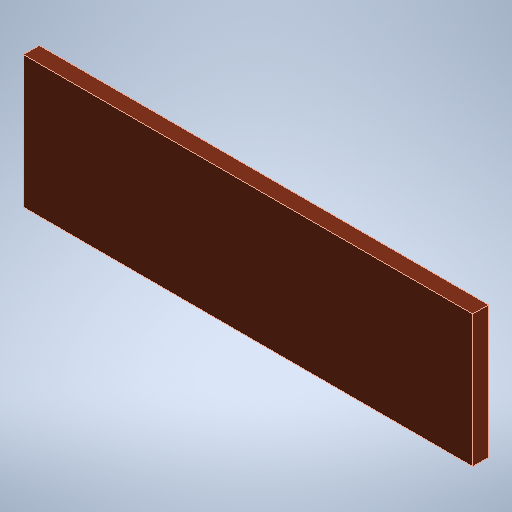
# Autodesk Inventor part: wall extension
Saved by Autodesk Inventor 2025.4 (Build 294407000, 407)
## iProperties
Created: 2026-04-19
Part Number: wall extension
Material: Generic
Document SubType Name: Modeling
Designer: lenovo
Density: 1 g/cm^3
Appearance: Default(1)
Author: lenovo
Autodesk Inventor part; units mm, degrees
ref_plane "YZ Plane" through (0, 0, 0) normal (1, 0, 0) x (0, 1, 0)
ref_plane "XZ Plane" through (0, 0, 0) normal (0, 1, 0) x (-1, 0, 0)
ref_plane "XY Plane" through (0, 0, 0) normal (0, 0, 1) x (1, 0, 0)
sketch "Sketch1" plane through (0, 0, 0) normal (0, 0, 1) x (1, 0, 0)
  line L0 (-42.5, -12.5) -> (42.5, -12.5)
  line L1 (42.5, -12.5) -> (42.5, 12.5)
  line L2 (42.5, 12.5) -> (-42.5, 12.5)
  line L3 (-42.5, 12.5) -> (-42.5, -12.5)
  line L4 (-42.5, -12.5) -> (42.5, 12.5) construction
  line L5 (42.5, -12.5) -> (-42.5, 12.5) construction
  point P0 (0, 0)
  dimension "d0" = 85
  dimension "d1" = 25
  constraints: 12 end point, 2 midpoint, 2 parallel, 1 horizontal, 1 perpendicular
  measures "d0" distance of L2.end L1.end
  measures "d1" distance of L1.end L0.end
extrude "Extrusion1" add sketch "Sketch1" along normal blind 3
body "Solid1"
